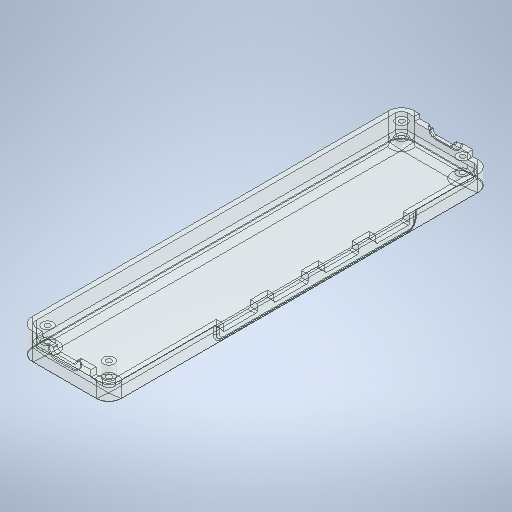
# Autodesk Inventor part: Upper_Housing
Saved by Autodesk Inventor 2025.1 (Build 291241020, 241B)
## iProperties
Created: 2026-01-18
Part Number: Upper_Housing
Material: Resina de poliariletercetona
Document SubType Name: Modeling
Designer: JoaoVitorRamosMitidi
Density: 1.32 g/cm^3
Appearance: Transparente
Mass: 26.3255 g
Surface Area: 155.575 cm^2
Volume: 19.9436 cm^3
Author: JoaoVitorRamosMitidi
Autodesk Inventor part; units mm, degrees
ref_plane "YZ Plane" through (0, 0, 0) normal (1, 0, 0) x (0, 1, 0)
ref_plane "XZ Plane" through (0, 0, 0) normal (0, 1, 0) x (-1, 0, 0)
ref_plane "XY Plane" through (0, 0, 0) normal (0, 0, 1) x (1, 0, 0)
sketch "Esboço1" plane through (0, 0, 0) normal (0, 1, 0) x (-1, 0, 0)
  line L0 (-12.5, 75) -> (12.5, 75)
  line L1 (17.5, 70) -> (17.5, -70)
  line L2 (12.5, -75) -> (-12.5, -75)
  line L3 (-17.5, -70) -> (-17.5, 70)
  line L4 (-17.5, 75) -> (17.5, -75) construction
  line L5 (17.5, 75) -> (-17.5, -75) construction
  line L6 (-13, 73) -> (13, 73)
  line L7 (15.5, 70.5) -> (15.5, -70.5)
  line L8 (13, -73) -> (-13, -73)
  line L9 (-15.5, -70.5) -> (-15.5, 70.5)
  line L10 (-15.5, 73) -> (15.5, -73) construction
  line L11 (15.5, 73) -> (-15.5, -73) construction
  circle A0 centre (12, 69.5) radius 1
  circle A1 centre (-12, 69.5) radius 1
  circle A2 centre (-12, -69.5) radius 1
  circle A3 centre (12, -69.5) radius 1
  line L12 (-11.2693, 48.2969) -> (11.2693, -48.2969) construction
  line L13 (11.6146, 48.7168) -> (-11.6146, -48.7168) construction
  line L14 (-13, 72.5) -> (13, 72.5)
  line L15 (15, 70.5) -> (15, -70.5)
  line L16 (13, -72.5) -> (-13, -72.5)
  line L17 (-15, -70.5) -> (-15, 70.5)
  line L18 (-15, 72.5) -> (15, -72.5) construction
  line L19 (15, 72.5) -> (-15, -72.5) construction
  arc A4 (-13, 72.5) -> (-15, 70.5) centre (-13, 70.5) ccw
  arc A5 (15, 70.5) -> (13, 72.5) centre (13, 70.5) ccw
  arc A6 (-15, -70.5) -> (-13, -72.5) centre (-13, -70.5) ccw
  arc A7 (13, -72.5) -> (15, -70.5) centre (13, -70.5) ccw
  arc A8 (-13, 73) -> (-15.5, 70.5) centre (-13, 70.5) ccw
  arc A9 (15.5, 70.5) -> (13, 73) centre (13, 70.5) ccw
  arc A10 (13, -73) -> (15.5, -70.5) centre (13, -70.5) ccw
  arc A11 (-15.5, -70.5) -> (-13, -73) centre (-13, -70.5) ccw
  arc A12 (-12.5, 75) -> (-17.5, 70) centre (-12.5, 70) ccw
  arc A13 (17.5, 70) -> (12.5, 75) centre (12.5, 70) ccw
  arc A14 (-17.5, -70) -> (-12.5, -75) centre (-12.5, -70) ccw
  arc A15 (12.5, -75) -> (17.5, -70) centre (12.5, -70) ccw
  circle A16 centre (-12, 69.5) radius 2.15
  circle A17 centre (12, 69.5) radius 2.15
  circle A18 centre (12, -69.5) radius 2.15
  circle A19 centre (-12, -69.5) radius 2.15
  line L20 (10.5, -75) -> (10.5, -73)
  line L21 (10.5, 73) -> (10.5, 75)
  line L22 (-10.5, -75) -> (-10.5, -73)
  line L23 (-10.5, 73) -> (-10.5, 75)
  point P0 (0, 0)
  dimension "d4" = 146
  dimension "d5" = 31
  dimension "d7" = 30
  dimension "d8" = 145
  dimension "d9" = 3
  dimension "d10" = 3
  dimension "d11" = 3
  dimension "d12" = 3
  dimension "d13" = 2
  dimension "d14" = 2
  dimension "d15" = 2.5
  dimension "d16" = 5
  dimension "d21" = 4.3
  dimension "d24" = 7
  dimension "d25" = 7
  dimension "d28" = 7
  dimension "d29" = 7
  dimension "d32" = 2.5
  dimension "d33" = 2.5
  constraints: 48 end point, 33 point on line, 24 point on circle, 24 tangent, 20 centre point, 15 equal radius, 8 midpoint, 7 perpendicular, 6 parallel, 4 coincident, 3 horizontal, 2 horizontal alignment, 2 vertical alignment
  measures "d4" distance of L11.start L10.end
  measures "d5" distance of L10.start L11.start
  measures "d7" distance of L18.start L19.start
  measures "d8" distance of L19.start L18.end
  measures "d9" distance from line of L17 A1.centre
  measures "d10" distance from line of L14 A1.centre
  measures "d11" distance from line of L16 A3.centre
  measures "d12" distance from line of L15 A3.centre
  measures "d13" diameter of A3
  measures "d14" radius of A4
  measures "d15" radius of A8
  measures "d16" radius of A12
  measures "d21" diameter of A19
  measures "d24" distance between parallel lines of L1 L20
  measures "d25" distance between parallel lines of L1 L21
  measures "d28" distance between parallel lines of L3 L23
  measures "d29" distance between parallel lines of L3 L22
  measures "d32" distance between parallel lines of L1 L15
  measures "d33" distance between parallel lines of L14 L0
extrude "Extrusão1" add sketch "Esboço1" along normal blind 3 contours L6 A9 L7 A10 L8 A11 L9 A8 | L14 A5 L15 A7 L16 A6 L17 A4 | A16 | A17 | A18 | A19
extrude "Extrusão2" add sketch "Esboço1" along normal blind 10.463 contours A16 | A17 | A18 | A19
extrude "Extrusão3" add sketch "Esboço1" along normal blind 3 contours L0 L23 L6 A8 L9 A11 L8 L22 L2 A14 L3 A12 | L0 L21 L6 L23 | L0 A13 L1 A15 L2 L20 L8 A10 L7 A9 L6 L21 | L22 L8 L20 L2
extrude "Extrusão5" add sketch "Esboço1" along normal blind 6.86 contours L0 L23 L6 A8 L9 A11 L8 L22 L2 A14 L3 A12
sketch "Esboço2" plane through (17.5, 0, 70) normal (1, 0, 0) x (0, 0, -1)
  line L0 (0, 6.86) -> (140, 6.86) projected
  line L1 (112.63, 6.86) -> (112.63, 4.485)
  line L2 (111.98, 3.835) -> (99.88, 3.835)
  line L3 (99.23, 4.485) -> (99.23, 6.86)
  line L4 (92.63, 6.86) -> (92.63, 4.485)
  line L5 (91.98, 3.835) -> (79.88, 3.835)
  line L6 (79.23, 4.485) -> (79.23, 6.86)
  line L7 (72.63, 6.86) -> (72.63, 4.485)
  line L8 (71.98, 3.835) -> (59.88, 3.835)
  line L9 (59.23, 4.485) -> (59.23, 6.86)
  line L10 (52.63, 6.86) -> (52.63, 4.485)
  line L11 (51.98, 3.835) -> (39.88, 3.835)
  line L12 (39.23, 4.485) -> (39.23, 6.86)
  line L13 (0, 0) -> (140, 0) projected
  line L14 (145, 0) -> (145, 6.86) projected
  line L15 (-5, 0) -> (-5, 6.86) projected
  arc A0 (111.98, 3.835) -> (112.63, 4.485) centre (111.98, 4.485) ccw
  arc A1 (99.23, 4.485) -> (99.88, 3.835) centre (99.88, 4.485) ccw
  arc A2 (91.98, 3.835) -> (92.63, 4.485) centre (91.98, 4.485) ccw
  arc A3 (79.23, 4.485) -> (79.88, 3.835) centre (79.88, 4.485) ccw
  arc A4 (71.98, 3.835) -> (72.63, 4.485) centre (71.98, 4.485) ccw
  arc A5 (59.23, 4.485) -> (59.88, 3.835) centre (59.88, 4.485) ccw
  arc A6 (51.98, 3.835) -> (52.63, 4.485) centre (51.98, 4.485) ccw
  arc A7 (39.23, 4.485) -> (39.88, 3.835) centre (39.88, 4.485) ccw
  point P0 (70, 0)
  point P1 (99.23, 3.835)
  point P2 (92.63, 3.835)
  point P3 (79.23, 3.835)
  point P4 (72.63, 3.835)
  point P5 (59.23, 3.835)
  point P6 (52.63, 3.835)
  point P7 (92.63, 5.6725)
  point P8 (52.63, 5.6725)
  point P9 (59.23, 5.6725)
  dimension "d34" = 3.835
  dimension "d35" = 13.4
  dimension "d36" = 6.6
  dimension "d37" = 6.6
  dimension "d38" = 6.6
  dimension "d39" = 32.37
  dimension "d40" = 44.23
  dimension "d41" = 0.65
  constraints: 24 end point, 16 point on circle, 16 tangent, 12 point on line, 8 centre point, 7 equal radius, 7 vertical, 5 perpendicular, 3 collinear, 3 horizontal alignment, 3 midpoint, 9 other
  measures "d34" distance between parallel lines of L13 L2
  measures "d35" distance between parallel lines of L3 L1
  measures "d36" distance from line of point (92.63, 5.672) L3
  measures "d37" distance between parallel lines of L7 L6
  measures "d38" distance of point (52.63, 5.672) point (59.23, 5.672)
  measures "d39" distance between parallel lines of L14 L1
  measures "d40" distance between parallel lines of L15 L12
  measures "d41" radius of A0
extrude "Extrusão6" cut sketch "Esboço2" against normal up to surface (2 mm away)
extrude "Extrusão7" add sketch "Esboço1" along normal blind 9.35 contours L0 L21 L6 L23
sketch "Esboço3" plane through (-12.5, 0, 75) normal (0, 0, 1) x (1, 0, 0)
  line L0 (2, 9.35) -> (23, 9.35) projected
  line L1 (17.108, 9.35) -> (17.108, 8.975)
  line L2 (15.658, 7.525) -> (9.318, 7.525)
  line L3 (7.868, 8.975) -> (7.868, 9.35)
  line L4 (0, 0) -> (25, 0) projected
  line L5 (30, 0) -> (30, 6.86) projected
  line L6 (-5, 0) -> (-5, 3) projected
  arc A0 (15.658, 7.525) -> (17.108, 8.975) centre (15.658, 8.975) ccw
  arc A1 (7.868, 8.975) -> (9.318, 7.525) centre (9.318, 8.975) ccw
  point P0 (12.5, 0)
  point P1 (17.108, 7.525)
  point P2 (7.868, 7.525)
  point P3 (7.868, 9.1625)
  dimension "d46" = 9.24
  dimension "d47" = 7.525
  dimension "d48" = 12.892
  dimension "d49" = 12.868
  dimension "d50" = 1.45
  constraints: 6 end point, 6 point on line, 4 point on circle, 4 tangent, 3 perpendicular, 2 centre point, 1 equal radius, 1 midpoint
  measures "d46" distance of point (17.108, 7.525) point (7.868, 7.525)
  measures "d47" distance between parallel lines of L4 L2
  measures "d48" distance between parallel lines of L5 L1
  measures "d49" distance from line of L6 point (7.868, 9.163)
  measures "d50" radius of A0
extrude "Extrusão8" cut sketch "Esboço3" against normal up to surface (2 mm away)
extrude "Extrusão9" add sketch "Esboço1" along normal blind 9.275 contours L22 L8 L20 L2
sketch "Esboço4" plane through (12.5, 0, -75) normal (0, 0, -1) x (-1, 0, 0)
  line L0 (23, 9.275) -> (2, 9.275) projected
  line L1 (17.12, 9.275) -> (17.12, 9.085)
  line L2 (15.67, 7.635) -> (9.33, 7.635)
  line L3 (7.88, 9.085) -> (7.88, 9.275)
  line L4 (0, 0) -> (25, 0) projected
  line L5 (30, 0) -> (30, 3) projected
  line L6 (-5, 0) -> (-5, 6.86) projected
  arc A0 (15.67, 7.635) -> (17.12, 9.085) centre (15.67, 9.085) ccw
  arc A1 (7.88, 9.085) -> (9.33, 7.635) centre (9.33, 9.085) ccw
  point P0 (12.5, 0)
  point P1 (17.12, 7.635)
  point P2 (7.88, 7.635)
  point P3 (12.5, 7.635)
  dimension "d55" = 9.24
  dimension "d56" = 7.635
  dimension "d57" = 12.88
  dimension "d58" = 12.88
  dimension "d59" = 1.45
  constraints: 6 end point, 6 point on line, 4 point on circle, 4 tangent, 2 centre point, 2 perpendicular, 1 equal radius, 1 midpoint, 1 vertical
  measures "d55" distance of point (17.12, 7.635) point (7.88, 7.635)
  measures "d56" distance from line of L4 point (12.5, 7.635)
  measures "d57" distance between parallel lines of L5 L1
  measures "d58" distance between parallel lines of L6 L3
  measures "d59" radius of A0
extrude "Extrusão10" cut sketch "Esboço4" against normal up to surface (2 mm away)
extrude "Extrusão11" add sketch "Esboço1" along normal blind 10.963 contours L0 A13 L1 A15 L2 L20 L8 A10 L7 A9 L6 L21
extrude "Extrusão12" add sketch "Esboço1" along normal blind 5 contours A0 | A1 | A2 | A3
thread "Rosca1" size "M2x0.4" class "6H" standard "ANSI Metric M Profile" full length
thread "Rosca2" size "M2x0.4" class "6H" standard "ANSI Metric M Profile" full length
thread "Rosca3" size "M2x0.4" class "6H" standard "ANSI Metric M Profile" full length
thread "Rosca4" size "M2x0.4" class "6H" standard "ANSI Metric M Profile" full length
fillet "Arredondamento1" radius 2 12 edges at (-14.7678, 3, -72.2678) (-15.5, 3, 0) (-14.7678, 3, 72.2678) (0, 3, 73) (14.7678, 3, 72.2678) (15.5, 3, 0) (14.7678, 3, -72.2678) (0, 3, -73) (14.15, 3, -69.5) (-9.85, 3, -69.5) (-9.85, 3, 69.5) (14.15, 3, 69.5)
sketch "Esboço6" plane through (17.5, 0, 70) normal (1, 0, 0) x (0, 0, -1)
  line L0 (59.23, 4.485) -> (59.23, 6.86) projected
  line L1 (52.63, 6.86) -> (59.23, 6.86) projected
  line L2 (52.63, 6.86) -> (52.63, 4.485) projected
  arc A0 (51.98, 3.835) -> (52.63, 4.485) centre (51.98, 4.485) ccw projected
  line L3 (51.98, 3.835) -> (39.88, 3.835) projected
  arc A1 (39.23, 4.485) -> (39.88, 3.835) centre (39.88, 4.485) ccw projected
  line L4 (39.23, 4.485) -> (39.23, 6.86) projected
  line L5 (0, 6.86) -> (39.23, 6.86) projected
  line L6 (0, 0) -> (0, 6.86) projected
  line L7 (0, 0) -> (140, 0) projected
  line L8 (140, 0) -> (140, 6.86) projected
  line L9 (112.63, 6.86) -> (140, 6.86) projected
  line L10 (112.63, 6.86) -> (112.63, 4.485) projected
  arc A2 (111.98, 3.835) -> (112.63, 4.485) centre (111.98, 4.485) ccw projected
  line L11 (111.98, 3.835) -> (99.88, 3.835) projected
  arc A3 (99.23, 4.485) -> (99.88, 3.835) centre (99.88, 4.485) ccw projected
  line L12 (99.23, 4.485) -> (99.23, 6.86) projected
  line L13 (92.63, 6.86) -> (99.23, 6.86) projected
  line L14 (92.63, 6.86) -> (92.63, 4.485) projected
  arc A4 (91.98, 3.835) -> (92.63, 4.485) centre (91.98, 4.485) ccw projected
  line L15 (91.98, 3.835) -> (79.88, 3.835) projected
  arc A5 (79.23, 4.485) -> (79.88, 3.835) centre (79.88, 4.485) ccw projected
  line L16 (79.23, 4.485) -> (79.23, 6.86) projected
  line L17 (72.63, 6.86) -> (79.23, 6.86) projected
  line L18 (72.63, 6.86) -> (72.63, 4.485) projected
  arc A6 (71.98, 3.835) -> (72.63, 4.485) centre (71.98, 4.485) ccw projected
  line L19 (71.98, 3.835) -> (59.88, 3.835) projected
  arc A7 (59.23, 4.485) -> (59.88, 3.835) centre (59.88, 4.485) ccw projected
  line L20 (114.63, 6.86) -> (114.63, 4.16)
  line L21 (112.305, 1.835) -> (39.555, 1.835)
  line L22 (37.23, 4.16) -> (37.23, 6.86)
  arc A8 (37.23, 4.16) -> (39.555, 1.835) centre (39.555, 4.16) ccw
  arc A9 (112.305, 1.835) -> (114.63, 4.16) centre (112.305, 4.16) ccw
  point P0 (70, 0)
  dimension "d80" = 2
  dimension "d81" = 2
  dimension "d82" = 2
  dimension "d83" = 2.325
  constraints: 6 end point, 4 point on circle, 4 tangent, 2 centre point, 2 perpendicular, 2 point on line, 1 equal radius, 1 vertical
  measures "d80" distance between parallel lines of L10 L20
  measures "d81" distance between parallel lines of L21 L11
  measures "d82" distance between parallel lines of L22 L4
  measures "d83" radius of A8
extrude "Extrusão13" add sketch "Esboço6" along normal blind 0.65 contours A7 L19 A6 L18 L17 L16 A5 L15 A4 L14 L13 L12 A3 L11 A2 L10 L9 L20 A9 L21 A8 L22 L5 L4 A1 L3 A0 L2 L1 L0
chamfer "Chanfro2" distance 0.65 angle 45 15 edges at (17.5, 5.51, -44.63) (17.5, 3.9971, -44.6243) (17.5, 2.516, -43.949) (17.5, 1.8407, -42.4679) (17.5, 1.835, -35.7675) (17.5, 1.835, -25.93) (17.5, 1.835, -15.93) (17.5, 1.835, -5.93) (17.5, 1.835, 4.07) (17.5, 1.835, 14.07) (17.5, 1.835, 23.9075) (17.5, 1.8407, 30.6079) (17.5, 2.516, 32.089) (17.5, 3.9971, 32.7643) (17.5, 5.51, 32.77)
fillet "Arredondamento4" radius 1 10 edges at (18.15, 2.516, -43.949) (18.15, 1.835, -5.93) (18.15, 2.516, 32.089) (18.15, 5.51, 32.77) (18.15, 5.51, -44.63) (17.5, 2.0564, -44.4086) (17.5, 1.185, -5.93) (17.5, 2.0564, 32.5486) (17.5, 5.51, 33.42) (17.5, 5.51, -45.28)
chamfer "Chanfro3" distance 5 distance2 0.5 8 edges at (17.5, 0, 0) (16.0355, 0, -73.5355) (0, 0, -75) (-16.0355, 0, -73.5355) (-17.5, 0, 0) (-16.0355, 0, 73.5355) (0, 0, 75) (16.0355, 0, 73.5355) measured on face at (-15.682, 0, 73.182) measured on face at (0, 0, 74.5) measured on face at (0, 0, -74.5) measured on face at (15.682, 0, -73.182) measured on face at (-15.682, 0, -73.182) measured on face at (17, 0, 0) measured on face at (15.682, 0, 73.182) measured on face at (-17, 0, 0)
fillet "Arredondamento5" radius 0.2 8 edges at (16.0355, 0.4999, 73.5355) (0, 0.4999, 75) (-16.0355, 0.4999, 73.5355) (-17.5, 0.4999, 0) (-16.0355, 0.4999, -73.5355) (0, 0.4999, -75) (16.0355, 0.4999, -73.5355) (17.5, 0.4999, 0)
sketch "Esboço10" plane through (12.5, 6.86, -75) normal (0, 0, -1) x (-1, 0, 0)
  line L0 (25, -6.179) -> (0, -6.179) projected
  line L1 (25, -6.179) -> (25, 4.103) projected
  line L2 (23, 4.103) -> (25, 4.103) projected
  line L3 (23, 2.415) -> (23, 4.103) projected
  line L4 (17.12, 2.415) -> (23, 2.415) projected
  line L5 (17.12, 2.415) -> (17.12, 2.225) projected
  arc A0 (15.67, 0.775) -> (17.12, 2.225) centre (15.67, 2.225) ccw projected
  line L6 (15.67, 0.775) -> (9.33, 0.775) projected
  arc A1 (7.88, 2.225) -> (9.33, 0.775) centre (9.33, 2.225) ccw projected
  line L7 (7.88, 2.225) -> (7.88, 2.415) projected
  line L8 (2, 2.415) -> (7.88, 2.415) projected
  line L9 (2, 0) -> (2, 2.415) projected
  line L10 (0, 0) -> (2, 0) projected
  line L11 (0, -6.179) -> (0, 0) projected
  line L12 (6.13, 2.415) -> (6.13, 2.225)
  line L13 (9.33, -0.975) -> (15.67, -0.975)
  line L14 (18.87, 2.225) -> (18.87, 2.415)
  arc A2 (15.67, -0.975) -> (18.87, 2.225) centre (15.67, 2.225) ccw
  arc A3 (6.13, 2.225) -> (9.33, -0.975) centre (9.33, 2.225) ccw
  point P0 (12.5, -6.86)
  point P1 (17.12, 2.32)
  dimension "d97" = 1.75
  dimension "d98" = 1.75
  dimension "d99" = 1.75
  dimension "d100" = 3.2
  constraints: 6 end point, 4 point on circle, 4 tangent, 2 centre point, 2 perpendicular, 2 point on line, 1 equal radius, 1 midpoint, 1 vertical
  measures "d97" distance from line of point (17.12, 2.32) L14
  measures "d98" distance from line of L7.end L12
  measures "d99" distance between parallel lines of L13 L6
  measures "d100" radius of A2
extrude "Extrusão14" cut sketch "Esboço10" against normal blind 0.52 contours L14 A2 L13 A3 L12 L8 L7 A1 L6 A0 L5 L4
sketch "Esboço11" plane through (10.5, 6.86, 75) normal (0, 0, 1) x (1, 0, 0)
  line L0 (2, -6.179) -> (-23, -6.179) projected
  line L1 (2, -6.179) -> (2, 0) projected
  line L2 (0, 0) -> (2, 0) projected
  line L3 (0, 0) -> (0, 2.49) projected
  line L4 (-5.892, 2.49) -> (0, 2.49) projected
  line L5 (-5.892, 2.49) -> (-5.892, 2.115) projected
  arc A0 (-7.342, 0.665) -> (-5.892, 2.115) centre (-7.342, 2.115) ccw projected
  line L6 (-7.342, 0.665) -> (-13.682, 0.665) projected
  arc A1 (-15.132, 2.115) -> (-13.682, 0.665) centre (-13.682, 2.115) ccw projected
  line L7 (-15.132, 2.115) -> (-15.132, 2.49) projected
  line L8 (-21, 2.49) -> (-15.132, 2.49) projected
  line L9 (-21, 2.49) -> (-21, 4.103) projected
  line L10 (-23, 4.103) -> (-21, 4.103) projected
  line L11 (-23, -6.179) -> (-23, 4.103) projected
  line L12 (0, 2.49) -> (-5.892, 2.49) projected
  line L13 (-4.142, 2.49) -> (-4.142, 2.115)
  line L14 (-7.342, -1.085) -> (-13.682, -1.085)
  line L15 (-16.882, 2.115) -> (-16.882, 2.49)
  arc A2 (-7.342, -1.085) -> (-4.142, 2.115) centre (-7.342, 2.115) ccw
  arc A3 (-16.882, 2.115) -> (-13.682, -1.085) centre (-13.682, 2.115) ccw
  point P0 (-10.5, -6.86)
  point P1 (-15.132, 2.3025)
  dimension "d103" = 1.75
  dimension "d104" = 1.75
  dimension "d105" = 1.75
  dimension "d106" = 3.2
  constraints: 6 end point, 4 point on circle, 4 tangent, 3 perpendicular, 2 centre point, 2 point on line, 1 equal radius, 1 midpoint
  measures "d103" distance from line of point (-15.132, 2.303) L15
  measures "d104" distance between parallel lines of L5 L13
  measures "d105" distance between parallel lines of L6 L14
  measures "d106" radius of A2
extrude "Extrusão15" cut sketch "Esboço11" against normal blind 0.52 contours L13 A2 L14 A3 L15 L8 L7 A1 L6 A0 L5 L4
